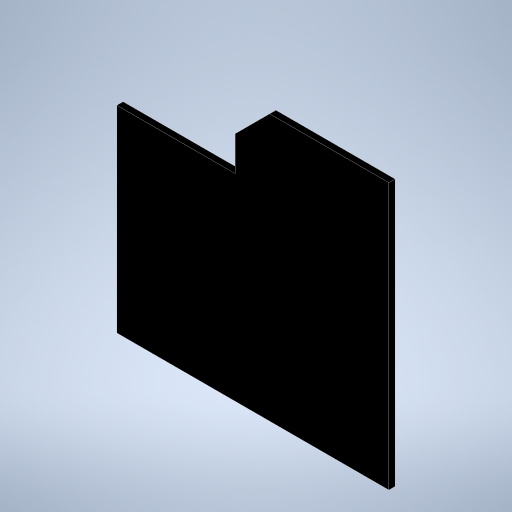
# Autodesk Inventor part: skimmer_swabbie_v1_BOARD
Saved by Autodesk Inventor 2023.2 (Build 272271000, 271)
## iProperties
Created: 2023-03-08
Part Number: skimmer_swabbie_v1_BOARD
Material: Generic
Document SubType Name: Modeling
Designer: atrus
Density: 1 g/cm^3
Appearance: BoardColor
Author: atrus
Autodesk Inventor part; units mm, degrees
ref_plane "YZ Plane" through (0, 0, 0) normal (1, 0, 0) x (0, 1, 0)
ref_plane "XZ Plane" through (0, 0, 0) normal (0, 1, 0) x (-1, 0, 0)
ref_plane "XY Plane" through (0, 0, 0) normal (0, 0, 1) x (1, 0, 0)
ref_plane "BoardFrontPlane" through (0, 0, 0) normal (0, 0, 1) x (1, 0, 0)
sketch "Sketch1" plane through (0, 0, 0) normal (0, 0, 1) x (1, 0, 0)
  line L0 (43.18, 34.29) -> (43.18, 85.09)
  line L1 (43.18, 85.09) -> (73.66, 85.09)
  line L2 (73.66, 85.09) -> (73.66, 93.98)
  line L3 (73.66, 93.98) -> (82.55, 102.87)
  line L4 (82.55, 102.87) -> (113.284, 102.87)
  line L5 (113.284, 102.87) -> (113.284, 34.29)
  line L6 (113.284, 34.29) -> (43.18, 34.29)
  constraints: 14 end point
extrude "BoardOutline" add sketch "Sketch1" along normal blind 1.6194
body "Solid1"
